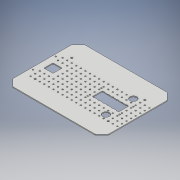
# Autodesk Inventor part: baseUp
Saved by Autodesk Inventor 2019.1 (Build 231200000, 200)
## iProperties
Created: 2018-05-21
Part Number: baseUp
Material: Типовые
Document SubType Name: Modeling
Designer: olege
Density: 1 g/cm^3
Appearance: По умолчанию
Mass: 63.0766 g
Surface Area: 659.094 cm^2
Volume: 63.0766 cm^3
Author: olege
Autodesk Inventor part; units mm, degrees
ref_plane "YZ Plane" through (0, 0, 0) normal (1, 0, 0) x (0, 1, 0)
ref_plane "XZ Plane" through (0, 0, 0) normal (0, 1, 0) x (-1, 0, 0)
ref_plane "XY Plane" through (0, 0, 0) normal (0, 0, 1) x (1, 0, 0)
sketch "Эскиз1" plane through (0, 0, 0) normal (0, 0, 1) x (1, 0, 0)
  line L0 (105, -79) -> (-105, -79)
  line L1 (-105, -79) -> (-105, 79)
  line L2 (-105, 79) -> (105, 79)
  line L3 (105, 79) -> (105, -79)
  line L4 (105, -79) -> (-105, 79) construction
  line L5 (-105, -79) -> (105, 79) construction
  point P0 (0, 0)
  dimension "d0" = 210
  dimension "d1" = 158
  constraints: 12 end point, 2 midpoint, 2 parallel, 1 horizontal, 1 perpendicular
  measures "d0" distance of L1.end L2.end
  measures "d1" distance of L0.end L1.end
extrude "Выдавливание1" add sketch "Эскиз1" along normal blind 2
chamfer "Фаска1" distance 15 angle 45 4 edges at (105, -79, 1) (-105, -79, 1) (-105, 79, 1) (105, 79, 1)
fillet "Сопряжение1" radius 2 8 edges at (90, 79, 1) (105, 64, 1) (105, -64, 1) (90, -79, 1) (-90, -79, 1) (-105, -64, 1) (-90, 79, 1) (-105, 64, 1)
sketch "Эскиз2" plane through (0, 0, 2) normal (0, 0, 1) x (1, 0, 0)
  line L0 (-100, 40) -> (100, 40) construction
  line L1 (100, 40) -> (100, -40) construction
  line L2 (100, -40) -> (-100, -40) construction
  line L3 (-100, -40) -> (-100, 40) construction
  line L4 (-100, 40) -> (100, -40) construction
  line L5 (100, 40) -> (-100, -40) construction
  circle A0 centre (100, -40) radius 1.5
  point P0 (0, 0)
  dimension "d8" = 200
  dimension "d9" = 80
  dimension "d10" = 3
  constraints: 12 end point, 2 midpoint, 2 parallel, 1 centre point, 1 coincident, 1 horizontal, 1 perpendicular
  measures "d8" distance of L1.end L2.end
  measures "d9" distance of L0.end L1.end
  measures "d10" diameter of A0
extrude "фонарь" cut sketch "Эскиз2" against normal blind 2
sketch "Эскиз3" plane through (0, 0, 2) normal (0, 0, 1) x (1, 0, 0)
  line L0 (-90, 20) -> (90, 20) construction
  line L1 (90, 20) -> (90, -20) construction
  line L2 (90, -20) -> (-90, -20) construction
  line L3 (-90, -20) -> (-90, 20) construction
  line L4 (-90, 20) -> (90, -20) construction
  line L5 (90, 20) -> (-90, -20) construction
  circle A0 centre (90, -20) radius 1.5
  circle A1 centre (90, 20) radius 1.5
  point P0 (0, 0)
  dimension "d16" = 180
  dimension "d17" = 40
  dimension "d18" = 3
  dimension "d19" = 3
  constraints: 12 end point, 2 centre point, 2 coincident, 2 midpoint, 2 parallel, 1 horizontal, 1 perpendicular
  measures "d16" distance of L1.end L2.end
  measures "d17" distance of L0.end L1.end
  measures "d18" diameter of A0
  measures "d19" diameter of A1
extrude "камера" cut sketch "Эскиз3" against normal blind 2
sketch "Эскиз4" plane through (0, 0, 2) normal (0, 0, 1) x (1, 0, 0)
  line L0 (-80, 40) -> (80, 40) construction
  line L1 (80, 40) -> (80, -40) construction
  line L2 (80, -40) -> (-80, -40) construction
  line L3 (-80, -40) -> (-80, 40) construction
  line L4 (-80, 40) -> (80, -40) construction
  line L5 (80, 40) -> (-80, -40) construction
  circle A0 centre (80, -40) radius 2
  circle A1 centre (-80, -40) radius 2
  circle A2 centre (-80, 40) radius 2
  circle A3 centre (80, 40) radius 2
  point P0 (0, 0)
  dimension "d22" = 160
  dimension "d23" = 80
  dimension "d24" = 4
  dimension "d25" = 4
  dimension "d26" = 4
  dimension "d27" = 4
  constraints: 12 end point, 4 centre point, 4 coincident, 2 midpoint, 2 parallel, 1 horizontal, 1 perpendicular
  measures "d22" distance of L1.end L2.end
  measures "d23" distance of L0.end L1.end
  measures "d24" diameter of A0
  measures "d25" diameter of A1
  measures "d26" diameter of A2
  measures "d27" diameter of A3
extrude "крепление" cut sketch "Эскиз4" against normal blind 2
sketch "Эскиз8" plane through (0, 0, 0) normal (0, 0, -1) x (-1, 0, 0)
  line L0 (-100, -25) -> (100, -25) construction
  line L1 (100, -25) -> (100, 25) construction
  line L2 (100, 25) -> (-100, 25) construction
  line L3 (-100, 25) -> (-100, -25) construction
  line L4 (-100, -25) -> (100, 25) construction
  line L5 (100, -25) -> (-100, 25) construction
  circle A0 centre (100, 25) radius 1.5
  circle A1 centre (100, -25) radius 1.5
  point P0 (0, 0)
  dimension "d65" = 200
  dimension "d66" = 50
  dimension "d67" = 3
  dimension "d68" = 3
  constraints: 12 end point, 2 centre point, 2 coincident, 2 midpoint, 2 parallel, 1 horizontal, 1 perpendicular
  measures "d65" distance of L2.end L1.end
  measures "d66" distance of L1.end L0.end
  measures "d67" diameter of A0
  measures "d68" diameter of A1
extrude "Дисплей" cut sketch "Эскиз8" against normal blind 10
sketch "Эскиз9" plane through (0, 0, 0) normal (0, 0, -1) x (-1, 0, 0)
  line L0 (-24.5, -10.5) -> (-65.5, 10.5) construction
  line L1 (-65.5, -10.5) -> (-24.5, 10.5) construction
  line L2 (-10, -15) -> (-80, -15) construction
  line L3 (-80, -15) -> (-80, 15) construction
  line L4 (-80, 15) -> (-10, 15) construction
  line L5 (-10, 15) -> (-10, -15) construction
  line L6 (-10, -15) -> (-80, 15) construction
  line L7 (-80, -15) -> (-10, 15) construction
  circle A0 centre (-80, 40) radius 2 construction
  circle A1 centre (-80, 15) radius 1.5
  circle A2 centre (-80, -15) radius 1.5
  circle A3 centre (-10, -15) radius 1.5
  circle A4 centre (-10, 15) radius 1.5
  line L8 (-74, 10.5) -> (-16, 10.5)
  line L9 (-16, 10.5) -> (-16, -10.5)
  line L10 (-16, -10.5) -> (-74, -10.5)
  line L11 (-74, -10.5) -> (-74, 10.5)
  line L12 (-74, 10.5) -> (-16, -10.5) construction
  line L13 (-16, 10.5) -> (-74, -10.5) construction
  point P0 (0, 0)
  point P1 (-45, 0)
  point P2 (-45, 0)
  dimension "d71" = 41
  dimension "d72" = 21
  dimension "d73" = 70
  dimension "d74" = 30
  dimension "d75" = 0
  dimension "d76" = 3
  dimension "d77" = 3
  dimension "d78" = 3
  dimension "d79" = 3
  dimension "d82" = 41
  dimension "d157" = 58
  dimension "d158" = 21
  constraints: 28 end point, 7 midpoint, 4 centre point, 4 coincident, 4 parallel, 2 horizontal, 2 perpendicular, 1 horizontal alignment
  measures "d71" distance of L0.end L1.end
  measures "d72" distance of L1.start L0.end
  measures "d73" distance of L3.end L4.end
  measures "d74" distance of L2.end L3.end
  measures "d75" horizontal distance of A0.centre L3.end
  measures "d76" diameter of A1
  measures "d77" diameter of A2
  measures "d78" diameter of A3
  measures "d79" diameter of A4
  measures "d82" distance of L0.start L1.start
  measures "d157" distance of L9.end L10.end
  measures "d158" distance of L8.end L9.end
extrude "Серво" cut sketch "Эскиз9" against normal blind 10
sketch "Эскиз10" plane through (0, 0, 0) normal (0, 0, -1) x (-1, 0, 0)
  line L0 (91, -10) -> (71, -10)
  line L1 (71, -10) -> (71, 10)
  line L2 (71, 10) -> (91, 10)
  line L3 (91, 10) -> (91, -10)
  line L4 (91, -10) -> (71, 10) construction
  line L5 (71, -10) -> (91, 10) construction
  line L6 (105, -63.1716) -> (105, 63.1716) projected
  point P0 (0, 0)
  point P1 (81, 0)
  point P2 (81, 0)
  dimension "d88" = 20
  dimension "d89" = 20
  dimension "d90" = 14
  constraints: 12 end point, 3 midpoint, 2 parallel, 1 horizontal, 1 horizontal alignment, 1 perpendicular
  measures "d88" distance of L1.end L2.end
  measures "d89" distance of L0.end L1.end
  measures "d90" distance between parallel lines of L6 L3
extrude "Для кабелей" cut sketch "Эскиз10" against normal blind 10
fillet "Сопряжение3" radius 2 4 edges at (-71, 10, 1) (-71, -10, 1) (-91, -10, 1) (-91, 10, 1)
sketch "Эскиз14" plane through (0, 0, 0) normal (0, 0, -1) x (-1, 0, 0)
  circle A0 centre (-65, -30) radius 7.5
  circle A1 centre (-65, 30) radius 7.5
  circle A2 centre (-80, 15) radius 1.5 projected
  circle A3 centre (-80, -15) radius 1.5 projected
  point P0 (0, 0)
  dimension "d118" = 15
  dimension "d119" = 15
  dimension "d120" = 15
  dimension "d121" = 15
  dimension "d122" = 15
  dimension "d123" = 15
  constraints: 2 centre point
  measures "d118" diameter of A0
  measures "d119" diameter of A1
  measures "d120" horizontal distance of A2.centre A1.centre
  measures "d121" horizontal distance of A3.centre A0.centre
  measures "d122" horizontal distance of A3.centre A0.centre
  measures "d123" horizontal distance of A2.centre A1.centre
extrude "Для проводов" cut sketch "Эскиз14" against normal blind 2 contours A0 | A1
sketch "Эскиз19" plane through (0, 0, 2) normal (0, 0, 1) x (1, 0, 0)
  arc A0 (-73, -10) -> (-71, -8) centre (-73, -8) ccw projected
  line L0 (-71, 8) -> (-71, -8) projected
  arc A1 (-71, 8) -> (-73, 10) centre (-73, 8) ccw projected
  line L1 (-89, 10) -> (-73, 10) projected
  arc A2 (-89, 10) -> (-91, 8) centre (-89, 8) ccw projected
  line L2 (-91, -8) -> (-91, 8) projected
  arc A3 (-91, -8) -> (-89, -10) centre (-89, -8) ccw projected
  line L3 (-73, -10) -> (-89, -10) projected
  point P0 (0, 0)
pattern_linear "Прямоуг.массив1" count 20 spacing 10 along (-1, 0, 0) count 8 spacing 10 along (0, 1, 0) of "фонарь"
sketch "Эскиз18" plane through (0, 0, 2) normal (0, 0, 1) x (1, 0, 0)
  arc A0 (-81.5, -10) -> (-78.5, -10) centre (-80, -10) ccw projected
  arc A1 (-91, 1.118) -> (-91, -1.118) centre (-90, 0) ccw projected
  line L0 (-65, 15) -> (-95, 15)
  line L1 (-95, 15) -> (-95, -15)
  line L2 (-95, -15) -> (-65, -15)
  line L3 (-65, -15) -> (-65, 15)
  line L4 (-65, 15) -> (-95, -15) construction
  line L5 (-95, 15) -> (-65, -15) construction
  arc A2 (-91, -8) -> (-89, -10) centre (-89, -8) ccw projected
  line L6 (-73, -10) -> (-89, -10) projected
  line L7 (-91, -8) -> (-91, 8) projected
  arc A3 (-89, 10) -> (-91, 8) centre (-89, 8) ccw projected
  line L8 (-89, 10) -> (-73, 10) projected
  arc A4 (-71, 8) -> (-73, 10) centre (-73, 8) ccw projected
  line L9 (-71, 8) -> (-71, -8) projected
  arc A5 (-73, -10) -> (-71, -8) centre (-73, -8) ccw projected
  point P0 (0, 0)
  point P1 (-80, 0)
  point P2 (-80, 0)
  point P3 (-80, 0)
  dimension "d170" = 30
  dimension "d171" = 30
  constraints: 12 end point, 4 midpoint, 2 parallel, 1 horizontal, 1 horizontal alignment, 1 perpendicular, 1 vertical alignment
  measures "d170" distance of L0.end L1.end
  measures "d171" distance of L0.start L0.end
extrude "Выдавливание17" add sketch "Эскиз18" against normal blind 2 contours L6 A0 | A1 L7 | L3 L2 L1 L0
equation "\"d119\" = d118"
equation "\"d120\" = d121"
equation "\"d123\" = d122"
